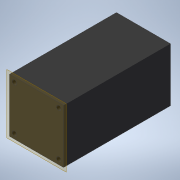
# Autodesk Inventor part: nema23
Saved by Autodesk Inventor 2020 (Build 240168000, 168)
## iProperties
Created: 2021-09-05
Part Number: nema23
Material: Generic
Document SubType Name: Modeling
Designer: super
Density: 1 g/cm^3
Appearance: Default
Author: super
Autodesk Inventor part; units mm, degrees
ref_plane "YZ Plane" through (0, 0, 0) normal (1, 0, 0) x (0, 1, 0)
ref_plane "XZ Plane" through (0, 0, 0) normal (0, 1, 0) x (-1, 0, 0)
sketch "Sketch1" plane through (0, 0, 0) normal (0, 0, 1) x (1, 0, 0)
  line L0 (0, 0) -> (57, 0)
  line L1 (57, 0) -> (57, 57)
  line L2 (57, 57) -> (0, 57)
  line L3 (0, 57) -> (0, 0)
  circle A0 centre (5, 5) radius 2.5
  circle A1 centre (52, 5) radius 2.5
  circle A2 centre (5, 52) radius 2.5
  circle A3 centre (52, 52) radius 2.5
  dimension "d0" = 57
  dimension "d1" = 57
  dimension "d2" = 5
  dimension "d3" = 5
  dimension "d4" = 5
  constraints: 8 end point, 4 centre point, 2 parallel, 1 horizontal, 1 perpendicular
  measures "d0" distance of L2.end L1.end
  measures "d1" distance of L1.end L0.end
  measures "d2" diameter of A0
  measures "d3" horizontal distance of L0.start A0.centre
  measures "d4" horizontal distance of L0.start A0.centre
extrude "Extrusion1" add sketch "Sketch1" against normal blind 113
body "Solid1"
